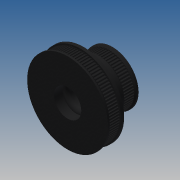
# Autodesk Inventor part: z idler pulley 3
Saved by Autodesk Inventor 2013 (Build 170138000, 138)
## iProperties
Created: 2017-04-05
Part Number: z idler pulley 3
Material: Generic
Document SubType Name: Modeling
Designer: employee
Density: 1 g/cm^3
Author: employee
Autodesk Inventor part; units mm, degrees
ref_plane "YZ Plane" through (0, 0, 0) normal (1, 0, 0) x (0, 1, 0)
ref_plane "XZ Plane" through (0, 0, 0) normal (0, 1, 0) x (-1, 0, 0)
ref_plane "XY Plane" through (0, 0, 0) normal (0, 0, 1) x (1, 0, 0)
sketch "Sketch1" plane through (0, 0, 0) normal (0, 1, 0) x (-1, 0, 0)
  circle A0 centre (0, 0) radius 31.577
  dimension "d0" = 63.154
  constraints: 1 centre point, 1 coincident
  measures "d0" diameter of A0
extrude "Extrusion1" add sketch "Sketch1" along normal mid plane 8
sketch "Sketch2" plane through (0, 4, 0) normal (0, 1, 0) x (1, 0, 0)
  circle A0 centre (0, 0) radius 31.577 projected
  circle A1 centre (0, 31.577) radius 0.795
  dimension "d5" = 1.59
  constraints: 2 vertical alignment, 1 centre point, 1 other
  measures "d5" diameter of A1
extrude "Extrusion2" cut sketch "Sketch2" against normal through all contours A1 A0 | A0 A1 picked at (0.0317, 31.3132) picked at (0.0304, 31.8395)
pattern_circular "Circular Pattern1" count 100 over 360 about axis through (0, 0, 0) along (0, 1, 0) of "Extrusion2"
sketch "Sketch4" plane through (0, -4, 0) normal (0, -1, 0) x (1, 0, 0)
  arc A0 (-31.1568, 5.1342) -> (-31.2184, 4.7451) centre (0, 0) ccw projected
  arc A1 (0.7949, -31.567) -> (1.1887, -31.5546) centre (0, 0) ccw projected
  circle A2 centre (0, 0) radius 32.577
  dimension "d12" = 1
  constraints: 1 centre point, 1 coincident
  measures "d12" radial gap between concentric circles of A0 A2
extrude "Extrusion3" add sketch "Sketch4" along normal blind 2.5
chamfer "Chamfer1" distance 1 angle 45 1 edges at (-32.577, -4, 0)
mirror "Mirror1" about plane through (0, 0, 0) normal (0, 1, 0) of "Extrusion3"
sketch "Sketch5" plane through (0, 6.5, 0) normal (0, 1, 0) x (1, 0, 0)
  circle A0 centre (0, 0) radius 32.577 projected
  circle A1 centre (0, 0) radius 20.1178
  dimension "d18" = 40.2357
  constraints: 1 centre point, 1 coincident
  measures "d18" diameter of A1
extrude "Extrusion4" add sketch "Sketch5" along normal blind 23.1 contours A1
sketch "Sketch6" plane through (0, 29.6, 0) normal (0, 1, 0) x (1, 0, 0)
  circle A0 centre (0, 0) radius 20.1178 projected
  circle A1 centre (0, 20.1178) radius 0.795
  dimension "d22" = 1.59
  constraints: 2 vertical alignment, 1 centre point, 1 other
  measures "d22" diameter of A1
extrude "Extrusion5" cut sketch "Sketch6" against normal up to surface (23.1 mm away) contours A1 A0 | A0 A1 picked at (0.0315, 19.8535) picked at (0.0295, 20.38)
pattern_circular "Circular Pattern2" count 64 over 360 about axis through (0, 6.5, 0) along (0, 1, 0) of "Extrusion5"
sketch "Sketch7" plane through (0, 6.5, 0) normal (0, 1, 0) x (1, 0, 0)
  arc A0 (3.1422, 19.8709) -> (2.7614, 19.9274) centre (0, 0) ccw projected
  arc A1 (3.1422, 19.8709) -> (4.7013, 19.5608) centre (3.9248, 19.7313) ccw projected
  arc A2 (5.0747, 19.4673) -> (4.7013, 19.5608) centre (0, 0) ccw projected
  arc A3 (5.0747, 19.4673) -> (6.596, 19.0058) centre (5.8399, 19.2516) ccw projected
  arc A4 (6.9584, 18.8761) -> (6.596, 19.0058) centre (0, 0) ccw projected
  arc A5 (6.9584, 18.8761) -> (8.4271, 18.2678) centre (7.6988, 18.5865) ccw projected
  arc A6 (8.7751, 18.1032) -> (8.4271, 18.2678) centre (0, 0) ccw projected
  arc A7 (8.7751, 18.1032) -> (10.1771, 17.3538) centre (9.4835, 17.7423) ccw projected
  arc A8 (10.5073, 17.1559) -> (10.1771, 17.3538) centre (0, 0) ccw projected
  arc A9 (10.5073, 17.1559) -> (11.829, 16.2727) centre (11.1769, 16.7274) ccw projected
  arc A10 (12.1382, 16.0434) -> (11.829, 16.2727) centre (0, 0) ccw projected
  arc A11 (12.1382, 16.0434) -> (13.3671, 15.0349) centre (12.7626, 15.5513) ccw projected
  arc A12 (13.6523, 14.7764) -> (13.3671, 15.0349) centre (0, 0) ccw projected
  arc A13 (13.6523, 14.7764) -> (14.7764, 13.6523) centre (14.2255, 14.2255) ccw projected
  arc A14 (15.0349, 13.3671) -> (14.7764, 13.6523) centre (0, 0) ccw projected
  arc A15 (15.0349, 13.3671) -> (16.0434, 12.1382) centre (15.5513, 12.7626) ccw projected
  arc A16 (16.2727, 11.829) -> (16.0434, 12.1382) centre (0, 0) ccw projected
  arc A17 (16.2727, 11.829) -> (17.1559, 10.5073) centre (16.7274, 11.1769) ccw projected
  arc A18 (17.3538, 10.1771) -> (17.1559, 10.5073) centre (0, 0) ccw projected
  arc A19 (17.3538, 10.1771) -> (18.1032, 8.7751) centre (17.7423, 9.4835) ccw projected
  arc A20 (18.2678, 8.4271) -> (18.1032, 8.7751) centre (0, 0) ccw projected
  arc A21 (18.2678, 8.4271) -> (18.8761, 6.9584) centre (18.5865, 7.6988) ccw projected
  arc A22 (19.0058, 6.596) -> (18.8761, 6.9584) centre (0, 0) ccw projected
  arc A23 (19.0058, 6.596) -> (19.4673, 5.0747) centre (19.2516, 5.8399) ccw projected
  arc A24 (19.5608, 4.7013) -> (19.4673, 5.0747) centre (0, 0) ccw projected
  arc A25 (19.5608, 4.7013) -> (19.8709, 3.1422) centre (19.7313, 3.9248) ccw projected
  arc A26 (19.9274, 2.7614) -> (19.8709, 3.1422) centre (0, 0) ccw projected
  arc A27 (19.9274, 2.7614) -> (20.0832, 1.1793) centre (20.021, 1.9719) ccw projected
  arc A28 (20.1021, 0.7948) -> (20.0832, 1.1793) centre (0, 0) ccw projected
  arc A29 (20.1021, 0.7948) -> (20.1021, -0.7948) centre (20.1178, 0) ccw projected
  arc A30 (20.0832, -1.1793) -> (20.1021, -0.7948) centre (0, 0) ccw projected
  arc A31 (20.0832, -1.1793) -> (19.9274, -2.7614) centre (20.021, -1.9719) ccw projected
  arc A32 (19.8709, -3.1422) -> (19.9274, -2.7614) centre (0, 0) ccw projected
  arc A33 (19.8709, -3.1422) -> (19.5608, -4.7013) centre (19.7313, -3.9248) ccw projected
  arc A34 (19.4673, -5.0747) -> (19.5608, -4.7013) centre (0, 0) ccw projected
  arc A35 (19.4673, -5.0747) -> (19.0058, -6.596) centre (19.2516, -5.8399) ccw projected
  arc A36 (18.8761, -6.9584) -> (19.0058, -6.596) centre (0, 0) ccw projected
  arc A37 (18.8761, -6.9584) -> (18.2678, -8.4271) centre (18.5865, -7.6988) ccw projected
  arc A38 (18.1032, -8.7751) -> (18.2678, -8.4271) centre (0, 0) ccw projected
  arc A39 (18.1032, -8.7751) -> (17.3538, -10.1771) centre (17.7423, -9.4835) ccw projected
  arc A40 (17.1559, -10.5073) -> (17.3538, -10.1771) centre (0, 0) ccw projected
  arc A41 (17.1559, -10.5073) -> (16.2727, -11.829) centre (16.7274, -11.1769) ccw projected
  arc A42 (16.0434, -12.1382) -> (16.2727, -11.829) centre (0, 0) ccw projected
  arc A43 (16.0434, -12.1382) -> (15.0349, -13.3671) centre (15.5513, -12.7626) ccw projected
  arc A44 (14.7764, -13.6523) -> (15.0349, -13.3671) centre (0, 0) ccw projected
  arc A45 (14.7764, -13.6523) -> (13.6523, -14.7764) centre (14.2255, -14.2255) ccw projected
  arc A46 (13.3671, -15.0349) -> (13.6523, -14.7764) centre (0, 0) ccw projected
  arc A47 (13.3671, -15.0349) -> (12.1382, -16.0434) centre (12.7626, -15.5513) ccw projected
  arc A48 (11.829, -16.2727) -> (12.1382, -16.0434) centre (0, 0) ccw projected
  arc A49 (11.829, -16.2727) -> (10.5073, -17.1559) centre (11.1769, -16.7274) ccw projected
  arc A50 (10.1771, -17.3538) -> (10.5073, -17.1559) centre (0, 0) ccw projected
  arc A51 (10.1771, -17.3538) -> (8.7751, -18.1032) centre (9.4835, -17.7423) ccw projected
  arc A52 (8.4271, -18.2678) -> (8.7751, -18.1032) centre (0, 0) ccw projected
  arc A53 (8.4271, -18.2678) -> (6.9584, -18.8761) centre (7.6988, -18.5865) ccw projected
  arc A54 (6.596, -19.0058) -> (6.9584, -18.8761) centre (0, 0) ccw projected
  arc A55 (6.596, -19.0058) -> (5.0747, -19.4673) centre (5.8399, -19.2516) ccw projected
  arc A56 (4.7013, -19.5608) -> (5.0747, -19.4673) centre (0, 0) ccw projected
  arc A57 (4.7013, -19.5608) -> (3.1422, -19.8709) centre (3.9248, -19.7313) ccw projected
  arc A58 (2.7614, -19.9274) -> (3.1422, -19.8709) centre (0, 0) ccw projected
  arc A59 (2.7614, -19.9274) -> (1.1793, -20.0832) centre (1.9719, -20.021) ccw projected
  arc A60 (0.7948, -20.1021) -> (1.1793, -20.0832) centre (0, 0) ccw projected
  arc A61 (0.7948, -20.1021) -> (-0.7948, -20.1021) centre (0, -20.1178) ccw projected
  arc A62 (-1.1793, -20.0832) -> (-0.7948, -20.1021) centre (0, 0) ccw projected
  arc A63 (-1.1793, -20.0832) -> (-2.7614, -19.9274) centre (-1.9719, -20.021) ccw projected
  arc A64 (-3.1422, -19.8709) -> (-2.7614, -19.9274) centre (0, 0) ccw projected
  arc A65 (-3.1422, -19.8709) -> (-4.7013, -19.5608) centre (-3.9248, -19.7313) ccw projected
  arc A66 (-5.0747, -19.4673) -> (-4.7013, -19.5608) centre (0, 0) ccw projected
  arc A67 (-5.0747, -19.4673) -> (-6.596, -19.0058) centre (-5.8399, -19.2516) ccw projected
  arc A68 (-6.9584, -18.8761) -> (-6.596, -19.0058) centre (0, 0) ccw projected
  arc A69 (-6.9584, -18.8761) -> (-8.4271, -18.2678) centre (-7.6988, -18.5865) ccw projected
  arc A70 (-8.7751, -18.1032) -> (-8.4271, -18.2678) centre (0, 0) ccw projected
  arc A71 (-8.7751, -18.1032) -> (-10.1771, -17.3538) centre (-9.4835, -17.7423) ccw projected
  arc A72 (-10.5073, -17.1559) -> (-10.1771, -17.3538) centre (0, 0) ccw projected
  arc A73 (-10.5073, -17.1559) -> (-11.829, -16.2727) centre (-11.1769, -16.7274) ccw projected
  arc A74 (-12.1382, -16.0434) -> (-11.829, -16.2727) centre (0, 0) ccw projected
  arc A75 (-12.1382, -16.0434) -> (-13.3671, -15.0349) centre (-12.7626, -15.5513) ccw projected
  arc A76 (-13.6523, -14.7764) -> (-13.3671, -15.0349) centre (0, 0) ccw projected
  arc A77 (-13.6523, -14.7764) -> (-14.7764, -13.6523) centre (-14.2255, -14.2255) ccw projected
  arc A78 (-15.0349, -13.3671) -> (-14.7764, -13.6523) centre (0, 0) ccw projected
  arc A79 (-15.0349, -13.3671) -> (-16.0434, -12.1382) centre (-15.5513, -12.7626) ccw projected
  arc A80 (-16.2727, -11.829) -> (-16.0434, -12.1382) centre (0, 0) ccw projected
  arc A81 (-16.2727, -11.829) -> (-17.1559, -10.5073) centre (-16.7274, -11.1769) ccw projected
  arc A82 (-17.3538, -10.1771) -> (-17.1559, -10.5073) centre (0, 0) ccw projected
  arc A83 (-17.3538, -10.1771) -> (-18.1032, -8.7751) centre (-17.7423, -9.4835) ccw projected
  arc A84 (-18.2678, -8.4271) -> (-18.1032, -8.7751) centre (0, 0) ccw projected
  arc A85 (-18.2678, -8.4271) -> (-18.8761, -6.9584) centre (-18.5865, -7.6988) ccw projected
  arc A86 (-19.0058, -6.596) -> (-18.8761, -6.9584) centre (0, 0) ccw projected
  arc A87 (-19.0058, -6.596) -> (-19.4673, -5.0747) centre (-19.2516, -5.8399) ccw projected
  arc A88 (-19.5608, -4.7013) -> (-19.4673, -5.0747) centre (0, 0) ccw projected
  arc A89 (-19.5608, -4.7013) -> (-19.8709, -3.1422) centre (-19.7313, -3.9248) ccw projected
  arc A90 (-19.9274, -2.7614) -> (-19.8709, -3.1422) centre (0, 0) ccw projected
  arc A91 (-19.9274, -2.7614) -> (-20.0832, -1.1793) centre (-20.021, -1.9719) ccw projected
  arc A92 (-20.1021, -0.7948) -> (-20.0832, -1.1793) centre (0, 0) ccw projected
  arc A93 (-20.1021, -0.7948) -> (-20.1021, 0.7948) centre (-20.1178, 0) ccw projected
  arc A94 (-20.0832, 1.1793) -> (-20.1021, 0.7948) centre (0, 0) ccw projected
  arc A95 (-20.0832, 1.1793) -> (-19.9274, 2.7614) centre (-20.021, 1.9719) ccw projected
  arc A96 (-19.8709, 3.1422) -> (-19.9274, 2.7614) centre (0, 0) ccw projected
  arc A97 (-19.8709, 3.1422) -> (-19.5608, 4.7013) centre (-19.7313, 3.9248) ccw projected
  arc A98 (-19.4673, 5.0747) -> (-19.5608, 4.7013) centre (0, 0) ccw projected
  arc A99 (-19.4673, 5.0747) -> (-19.0058, 6.596) centre (-19.2516, 5.8399) ccw projected
  arc A100 (-18.8761, 6.9584) -> (-19.0058, 6.596) centre (0, 0) ccw projected
  arc A101 (-18.8761, 6.9584) -> (-18.2678, 8.4271) centre (-18.5865, 7.6988) ccw projected
  arc A102 (-18.1032, 8.7751) -> (-18.2678, 8.4271) centre (0, 0) ccw projected
  arc A103 (-18.1032, 8.7751) -> (-17.3538, 10.1771) centre (-17.7423, 9.4835) ccw projected
  arc A104 (-17.1559, 10.5073) -> (-17.3538, 10.1771) centre (0, 0) ccw projected
  arc A105 (-17.1559, 10.5073) -> (-16.2727, 11.829) centre (-16.7274, 11.1769) ccw projected
  arc A106 (-16.0434, 12.1382) -> (-16.2727, 11.829) centre (0, 0) ccw projected
  arc A107 (-16.0434, 12.1382) -> (-15.0349, 13.3671) centre (-15.5513, 12.7626) ccw projected
  arc A108 (-14.7764, 13.6523) -> (-15.0349, 13.3671) centre (0, 0) ccw projected
  arc A109 (-14.7764, 13.6523) -> (-13.6523, 14.7764) centre (-14.2255, 14.2255) ccw projected
  arc A110 (-13.3671, 15.0349) -> (-13.6523, 14.7764) centre (0, 0) ccw projected
  arc A111 (-13.3671, 15.0349) -> (-12.1382, 16.0434) centre (-12.7626, 15.5513) ccw projected
  arc A112 (-11.829, 16.2727) -> (-12.1382, 16.0434) centre (0, 0) ccw projected
  arc A113 (-11.829, 16.2727) -> (-10.5073, 17.1559) centre (-11.1769, 16.7274) ccw projected
  arc A114 (-10.1771, 17.3538) -> (-10.5073, 17.1559) centre (0, 0) ccw projected
  arc A115 (-10.1771, 17.3538) -> (-8.7751, 18.1032) centre (-9.4835, 17.7423) ccw projected
  arc A116 (-8.4271, 18.2678) -> (-8.7751, 18.1032) centre (0, 0) ccw projected
  arc A117 (-8.4271, 18.2678) -> (-6.9584, 18.8761) centre (-7.6988, 18.5865) ccw projected
  arc A118 (-6.596, 19.0058) -> (-6.9584, 18.8761) centre (0, 0) ccw projected
  arc A119 (-6.596, 19.0058) -> (-5.0747, 19.4673) centre (-5.8399, 19.2516) ccw projected
  arc A120 (-4.7013, 19.5608) -> (-5.0747, 19.4673) centre (0, 0) ccw projected
  arc A121 (-4.7013, 19.5608) -> (-3.1422, 19.8709) centre (-3.9248, 19.7313) ccw projected
  arc A122 (-2.7614, 19.9274) -> (-3.1422, 19.8709) centre (0, 0) ccw projected
  arc A123 (-2.7614, 19.9274) -> (-1.1793, 20.0832) centre (-1.9719, 20.021) ccw projected
  arc A124 (-0.7948, 20.1021) -> (-1.1793, 20.0832) centre (0, 0) ccw projected
  arc A125 (-0.7948, 20.1021) -> (0.7948, 20.1021) centre (0, 20.1178) ccw projected
  arc A126 (1.1793, 20.0832) -> (0.7948, 20.1021) centre (0, 0) ccw projected
  arc A127 (1.1793, 20.0832) -> (2.7614, 19.9274) centre (1.9719, 20.021) ccw projected
  circle A128 centre (0, 0) radius 32.577 projected
  circle A129 centre (0, 0) radius 21.1178
  dimension "d29" = 1
  constraints: 1 centre point, 1 coincident
  measures "d29" radial gap between concentric circles of A98 A129
extrude "Extrusion6" add sketch "Sketch7" along normal blind 12.6 contours A129
sketch "Sketch8" plane through (0, 29.6, 0) normal (0, 1, 0) x (1, 0, 0)
  arc A0 (1.1793, 20.0832) -> (2.7614, 19.9274) centre (1.9719, 20.021) ccw projected
  arc A1 (1.1793, 20.0832) -> (0.7948, 20.1021) centre (0, 0) ccw projected
  arc A2 (-0.7948, 20.1021) -> (0.7948, 20.1021) centre (0, 20.1178) ccw projected
  arc A3 (-0.7948, 20.1021) -> (-1.1793, 20.0832) centre (0, 0) ccw projected
  arc A4 (-2.7614, 19.9274) -> (-1.1793, 20.0832) centre (-1.9719, 20.021) ccw projected
  arc A5 (-2.7614, 19.9274) -> (-3.1422, 19.8709) centre (0, 0) ccw projected
  arc A6 (-4.7013, 19.5608) -> (-3.1422, 19.8709) centre (-3.9248, 19.7313) ccw projected
  arc A7 (-4.7013, 19.5608) -> (-5.0747, 19.4673) centre (0, 0) ccw projected
  arc A8 (-6.596, 19.0058) -> (-5.0747, 19.4673) centre (-5.8399, 19.2516) ccw projected
  arc A9 (-6.596, 19.0058) -> (-6.9584, 18.8761) centre (0, 0) ccw projected
  arc A10 (-8.4271, 18.2678) -> (-6.9584, 18.8761) centre (-7.6988, 18.5865) ccw projected
  arc A11 (-8.4271, 18.2678) -> (-8.7751, 18.1032) centre (0, 0) ccw projected
  arc A12 (-10.1771, 17.3538) -> (-8.7751, 18.1032) centre (-9.4835, 17.7423) ccw projected
  arc A13 (-10.1771, 17.3538) -> (-10.5073, 17.1559) centre (0, 0) ccw projected
  arc A14 (-11.829, 16.2727) -> (-10.5073, 17.1559) centre (-11.1769, 16.7274) ccw projected
  arc A15 (-11.829, 16.2727) -> (-12.1382, 16.0434) centre (0, 0) ccw projected
  arc A16 (-13.3671, 15.0349) -> (-12.1382, 16.0434) centre (-12.7626, 15.5513) ccw projected
  arc A17 (-13.3671, 15.0349) -> (-13.6523, 14.7764) centre (0, 0) ccw projected
  arc A18 (-14.7764, 13.6523) -> (-13.6523, 14.7764) centre (-14.2255, 14.2255) ccw projected
  arc A19 (-14.7764, 13.6523) -> (-15.0349, 13.3671) centre (0, 0) ccw projected
  arc A20 (-16.0434, 12.1382) -> (-15.0349, 13.3671) centre (-15.5513, 12.7626) ccw projected
  arc A21 (-16.0434, 12.1382) -> (-16.2727, 11.829) centre (0, 0) ccw projected
  arc A22 (-17.1559, 10.5073) -> (-16.2727, 11.829) centre (-16.7274, 11.1769) ccw projected
  arc A23 (-17.1559, 10.5073) -> (-17.3538, 10.1771) centre (0, 0) ccw projected
  arc A24 (-18.1032, 8.7751) -> (-17.3538, 10.1771) centre (-17.7423, 9.4835) ccw projected
  arc A25 (-18.1032, 8.7751) -> (-18.2678, 8.4271) centre (0, 0) ccw projected
  arc A26 (-18.8761, 6.9584) -> (-18.2678, 8.4271) centre (-18.5865, 7.6988) ccw projected
  arc A27 (-18.8761, 6.9584) -> (-19.0058, 6.596) centre (0, 0) ccw projected
  arc A28 (-19.4673, 5.0747) -> (-19.0058, 6.596) centre (-19.2516, 5.8399) ccw projected
  arc A29 (-19.4673, 5.0747) -> (-19.5608, 4.7013) centre (0, 0) ccw projected
  arc A30 (-19.8709, 3.1422) -> (-19.5608, 4.7013) centre (-19.7313, 3.9248) ccw projected
  arc A31 (-19.8709, 3.1422) -> (-19.9274, 2.7614) centre (0, 0) ccw projected
  arc A32 (-20.0832, 1.1793) -> (-19.9274, 2.7614) centre (-20.021, 1.9719) ccw projected
  arc A33 (-20.0832, 1.1793) -> (-20.1021, 0.7948) centre (0, 0) ccw projected
  arc A34 (-20.1021, -0.7948) -> (-20.1021, 0.7948) centre (-20.1178, 0) ccw projected
  arc A35 (-20.1021, -0.7948) -> (-20.0832, -1.1793) centre (0, 0) ccw projected
  arc A36 (-19.9274, -2.7614) -> (-20.0832, -1.1793) centre (-20.021, -1.9719) ccw projected
  arc A37 (-19.9274, -2.7614) -> (-19.8709, -3.1422) centre (0, 0) ccw projected
  arc A38 (-19.5608, -4.7013) -> (-19.8709, -3.1422) centre (-19.7313, -3.9248) ccw projected
  arc A39 (-19.5608, -4.7013) -> (-19.4673, -5.0747) centre (0, 0) ccw projected
  arc A40 (-19.0058, -6.596) -> (-19.4673, -5.0747) centre (-19.2516, -5.8399) ccw projected
  arc A41 (-19.0058, -6.596) -> (-18.8761, -6.9584) centre (0, 0) ccw projected
  arc A42 (-18.2678, -8.4271) -> (-18.8761, -6.9584) centre (-18.5865, -7.6988) ccw projected
  arc A43 (-18.2678, -8.4271) -> (-18.1032, -8.7751) centre (0, 0) ccw projected
  arc A44 (-17.3538, -10.1771) -> (-18.1032, -8.7751) centre (-17.7423, -9.4835) ccw projected
  arc A45 (-17.3538, -10.1771) -> (-17.1559, -10.5073) centre (0, 0) ccw projected
  arc A46 (-16.2727, -11.829) -> (-17.1559, -10.5073) centre (-16.7274, -11.1769) ccw projected
  arc A47 (-16.2727, -11.829) -> (-16.0434, -12.1382) centre (0, 0) ccw projected
  arc A48 (-15.0349, -13.3671) -> (-16.0434, -12.1382) centre (-15.5513, -12.7626) ccw projected
  arc A49 (-15.0349, -13.3671) -> (-14.7764, -13.6523) centre (0, 0) ccw projected
  arc A50 (-13.6523, -14.7764) -> (-14.7764, -13.6523) centre (-14.2255, -14.2255) ccw projected
  arc A51 (-13.6523, -14.7764) -> (-13.3671, -15.0349) centre (0, 0) ccw projected
  arc A52 (-12.1382, -16.0434) -> (-13.3671, -15.0349) centre (-12.7626, -15.5513) ccw projected
  arc A53 (-12.1382, -16.0434) -> (-11.829, -16.2727) centre (0, 0) ccw projected
  arc A54 (-10.5073, -17.1559) -> (-11.829, -16.2727) centre (-11.1769, -16.7274) ccw projected
  arc A55 (-10.5073, -17.1559) -> (-10.1771, -17.3538) centre (0, 0) ccw projected
  arc A56 (-8.7751, -18.1032) -> (-10.1771, -17.3538) centre (-9.4835, -17.7423) ccw projected
  arc A57 (-8.7751, -18.1032) -> (-8.4271, -18.2678) centre (0, 0) ccw projected
  arc A58 (-6.9584, -18.8761) -> (-8.4271, -18.2678) centre (-7.6988, -18.5865) ccw projected
  arc A59 (-6.9584, -18.8761) -> (-6.596, -19.0058) centre (0, 0) ccw projected
  arc A60 (-5.0747, -19.4673) -> (-6.596, -19.0058) centre (-5.8399, -19.2516) ccw projected
  arc A61 (-5.0747, -19.4673) -> (-4.7013, -19.5608) centre (0, 0) ccw projected
  arc A62 (-3.1422, -19.8709) -> (-4.7013, -19.5608) centre (-3.9248, -19.7313) ccw projected
  arc A63 (-3.1422, -19.8709) -> (-2.7614, -19.9274) centre (0, 0) ccw projected
  arc A64 (-1.1793, -20.0832) -> (-2.7614, -19.9274) centre (-1.9719, -20.021) ccw projected
  arc A65 (-1.1793, -20.0832) -> (-0.7948, -20.1021) centre (0, 0) ccw projected
  arc A66 (0.7948, -20.1021) -> (-0.7948, -20.1021) centre (0, -20.1178) ccw projected
  arc A67 (0.7948, -20.1021) -> (1.1793, -20.0832) centre (0, 0) ccw projected
  arc A68 (2.7614, -19.9274) -> (1.1793, -20.0832) centre (1.9719, -20.021) ccw projected
  arc A69 (2.7614, -19.9274) -> (3.1422, -19.8709) centre (0, 0) ccw projected
  arc A70 (4.7013, -19.5608) -> (3.1422, -19.8709) centre (3.9248, -19.7313) ccw projected
  arc A71 (4.7013, -19.5608) -> (5.0747, -19.4673) centre (0, 0) ccw projected
  arc A72 (6.596, -19.0058) -> (5.0747, -19.4673) centre (5.8399, -19.2516) ccw projected
  arc A73 (6.596, -19.0058) -> (6.9584, -18.8761) centre (0, 0) ccw projected
  arc A74 (8.4271, -18.2678) -> (6.9584, -18.8761) centre (7.6988, -18.5865) ccw projected
  arc A75 (8.4271, -18.2678) -> (8.7751, -18.1032) centre (0, 0) ccw projected
  arc A76 (10.1771, -17.3538) -> (8.7751, -18.1032) centre (9.4835, -17.7423) ccw projected
  arc A77 (10.1771, -17.3538) -> (10.5073, -17.1559) centre (0, 0) ccw projected
  arc A78 (11.829, -16.2727) -> (10.5073, -17.1559) centre (11.1769, -16.7274) ccw projected
  arc A79 (11.829, -16.2727) -> (12.1382, -16.0434) centre (0, 0) ccw projected
  arc A80 (13.3671, -15.0349) -> (12.1382, -16.0434) centre (12.7626, -15.5513) ccw projected
  arc A81 (13.3671, -15.0349) -> (13.6523, -14.7764) centre (0, 0) ccw projected
  arc A82 (14.7764, -13.6523) -> (13.6523, -14.7764) centre (14.2255, -14.2255) ccw projected
  arc A83 (14.7764, -13.6523) -> (15.0349, -13.3671) centre (0, 0) ccw projected
  arc A84 (16.0434, -12.1382) -> (15.0349, -13.3671) centre (15.5513, -12.7626) ccw projected
  arc A85 (16.0434, -12.1382) -> (16.2727, -11.829) centre (0, 0) ccw projected
  arc A86 (17.1559, -10.5073) -> (16.2727, -11.829) centre (16.7274, -11.1769) ccw projected
  arc A87 (17.1559, -10.5073) -> (17.3538, -10.1771) centre (0, 0) ccw projected
  arc A88 (18.1032, -8.7751) -> (17.3538, -10.1771) centre (17.7423, -9.4835) ccw projected
  arc A89 (18.1032, -8.7751) -> (18.2678, -8.4271) centre (0, 0) ccw projected
  arc A90 (18.8761, -6.9584) -> (18.2678, -8.4271) centre (18.5865, -7.6988) ccw projected
  arc A91 (18.8761, -6.9584) -> (19.0058, -6.596) centre (0, 0) ccw projected
  arc A92 (19.4673, -5.0747) -> (19.0058, -6.596) centre (19.2516, -5.8399) ccw projected
  arc A93 (19.4673, -5.0747) -> (19.5608, -4.7013) centre (0, 0) ccw projected
  arc A94 (19.8709, -3.1422) -> (19.5608, -4.7013) centre (19.7313, -3.9248) ccw projected
  arc A95 (19.8709, -3.1422) -> (19.9274, -2.7614) centre (0, 0) ccw projected
  arc A96 (20.0832, -1.1793) -> (19.9274, -2.7614) centre (20.021, -1.9719) ccw projected
  arc A97 (20.0832, -1.1793) -> (20.1021, -0.7948) centre (0, 0) ccw projected
  arc A98 (20.1021, 0.7948) -> (20.1021, -0.7948) centre (20.1178, 0) ccw projected
  arc A99 (20.1021, 0.7948) -> (20.0832, 1.1793) centre (0, 0) ccw projected
  arc A100 (19.9274, 2.7614) -> (20.0832, 1.1793) centre (20.021, 1.9719) ccw projected
  arc A101 (19.9274, 2.7614) -> (19.8709, 3.1422) centre (0, 0) ccw projected
  arc A102 (19.5608, 4.7013) -> (19.8709, 3.1422) centre (19.7313, 3.9248) ccw projected
  arc A103 (19.5608, 4.7013) -> (19.4673, 5.0747) centre (0, 0) ccw projected
  arc A104 (19.0058, 6.596) -> (19.4673, 5.0747) centre (19.2516, 5.8399) ccw projected
  arc A105 (19.0058, 6.596) -> (18.8761, 6.9584) centre (0, 0) ccw projected
  arc A106 (18.2678, 8.4271) -> (18.8761, 6.9584) centre (18.5865, 7.6988) ccw projected
  arc A107 (18.2678, 8.4271) -> (18.1032, 8.7751) centre (0, 0) ccw projected
  arc A108 (17.3538, 10.1771) -> (18.1032, 8.7751) centre (17.7423, 9.4835) ccw projected
  arc A109 (17.3538, 10.1771) -> (17.1559, 10.5073) centre (0, 0) ccw projected
  arc A110 (16.2727, 11.829) -> (17.1559, 10.5073) centre (16.7274, 11.1769) ccw projected
  arc A111 (16.2727, 11.829) -> (16.0434, 12.1382) centre (0, 0) ccw projected
  arc A112 (15.0349, 13.3671) -> (16.0434, 12.1382) centre (15.5513, 12.7626) ccw projected
  arc A113 (15.0349, 13.3671) -> (14.7764, 13.6523) centre (0, 0) ccw projected
  arc A114 (13.6523, 14.7764) -> (14.7764, 13.6523) centre (14.2255, 14.2255) ccw projected
  arc A115 (13.6523, 14.7764) -> (13.3671, 15.0349) centre (0, 0) ccw projected
  arc A116 (12.1382, 16.0434) -> (13.3671, 15.0349) centre (12.7626, 15.5513) ccw projected
  arc A117 (12.1382, 16.0434) -> (11.829, 16.2727) centre (0, 0) ccw projected
  arc A118 (10.5073, 17.1559) -> (11.829, 16.2727) centre (11.1769, 16.7274) ccw projected
  arc A119 (10.5073, 17.1559) -> (10.1771, 17.3538) centre (0, 0) ccw projected
  arc A120 (8.7751, 18.1032) -> (10.1771, 17.3538) centre (9.4835, 17.7423) ccw projected
  arc A121 (8.7751, 18.1032) -> (8.4271, 18.2678) centre (0, 0) ccw projected
  arc A122 (6.9584, 18.8761) -> (8.4271, 18.2678) centre (7.6988, 18.5865) ccw projected
  arc A123 (6.9584, 18.8761) -> (6.596, 19.0058) centre (0, 0) ccw projected
  arc A124 (5.0747, 19.4673) -> (6.596, 19.0058) centre (5.8399, 19.2516) ccw projected
  arc A125 (5.0747, 19.4673) -> (4.7013, 19.5608) centre (0, 0) ccw projected
  arc A126 (3.1422, 19.8709) -> (4.7013, 19.5608) centre (3.9248, 19.7313) ccw projected
  arc A127 (3.1422, 19.8709) -> (2.7614, 19.9274) centre (0, 0) ccw projected
  circle A128 centre (0, 0) radius 21.1178 projected
extrude "Extrusion7" add sketch "Sketch8" against normal blind 2.5
chamfer "Chamfer2" distance 1 angle 45 2 edges at (-21.1178, 19.1, 0) (-21.1178, 27.1, 0)
sketch "Sketch9" plane through (0, 29.6, 0) normal (0, 1, 0) x (1, 0, 0)
  circle A0 centre (0, 0) radius 21.1178 projected
  circle A1 centre (0, 0) radius 7.5
  dimension "d37" = 15
  constraints: 1 centre point, 1 coincident
  measures "d37" diameter of A1
extrude "Extrusion8" cut sketch "Sketch9" against normal through all contours A1
sketch "Sketch10" plane through (0, 29.6, 0) normal (0, 1, 0) x (1, 0, 0)
  circle A0 centre (0, 0) radius 7.5 projected
  circle A1 centre (0, 0) radius 21.1178 projected
  circle A2 centre (0, 0) radius 11
  dimension "d41" = 22
  constraints: 1 centre point, 1 coincident
  measures "d41" diameter of A2
extrude "Extrusion9" cut sketch "Sketch10" against normal blind 7 contours A2
sketch "Sketch11" plane through (0, -6.5, 0) normal (0, -1, 0) x (1, 0, 0)
  circle A0 centre (0, 0) radius 7.5 projected
  circle A1 centre (0, 0) radius 32.577 projected
  circle A2 centre (0, 0) radius 11
  dimension "d45" = 22
  constraints: 1 centre point, 1 coincident
  measures "d45" diameter of A2
extrude "Extrusion10" cut sketch "Sketch11" against normal blind 7 contours A2
fillet "Fillet1" radius 3.5 2 edges at (-7.5, 0.5, 0) (-7.5, 22.6, 0)
body "Solid1"
